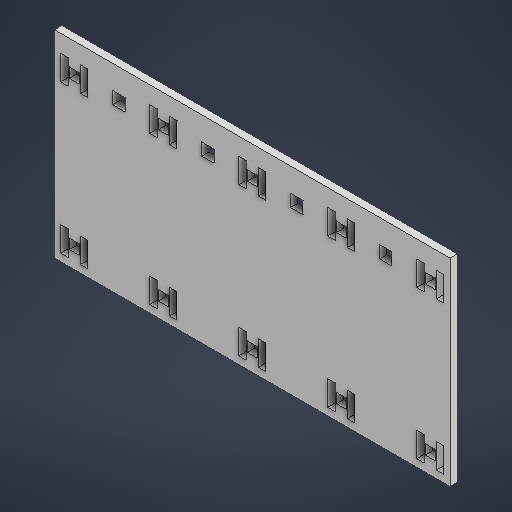
# Autodesk Inventor part: techo
Saved by Autodesk Inventor 2026 (Build 300175000, 175)
## iProperties
Created: 2026-05-15
Part Number: techo
Material: Generic
Document SubType Name: Modeling
Designer: juana
Density: 1 g/cm^3
Appearance: Default
Author: juana
Autodesk Inventor part; units mm, degrees
ref_plane "YZ Plane" through (0, 0, 0) normal (1, 0, 0) x (0, 1, 0)
ref_plane "XZ Plane" through (0, 0, 0) normal (0, 1, 0) x (-1, 0, 0)
ref_plane "XY Plane" through (0, 0, 0) normal (0, 0, 1) x (1, 0, 0)
sketch "Sketch1" plane through (0, 0, 0) normal (0, 0, 1) x (1, 0, 0)
  line L0 (0, 0) -> (160, 0)
  line L1 (160, 0) -> (160, 80)
  line L2 (160, 80) -> (0, 80)
  line L3 (0, 80) -> (0, 0)
  line L4 (2.5, 13) -> (5.5, 13)
  line L5 (5.5, 13) -> (5.5, 3)
  line L6 (5.5, 3) -> (2.5, 3)
  line L7 (2.5, 3) -> (2.5, 13)
  line L8 (10.5, 13) -> (13.5, 13)
  line L9 (13.5, 13) -> (13.5, 3)
  line L10 (13.5, 3) -> (10.5, 3)
  line L11 (10.5, 3) -> (10.5, 13)
  line L12 (0, 40) -> (160, 40) construction
  line L13 (80, 80) -> (80, 0) construction
  line L14 (0, 0) -> (0, 80)
  line L15 (2.5, 77) -> (2.5, 67) construction
  line L16 (13.5, 77) -> (10.5, 77)
  line L17 (157.5, 13) -> (154.5, 13)
  line L18 (154.5, 13) -> (154.5, 3)
  line L19 (154.5, 3) -> (157.5, 3)
  line L20 (157.5, 3) -> (157.5, 13)
  line L21 (149.5, 13) -> (146.5, 13)
  line L22 (146.5, 13) -> (146.5, 3)
  line L23 (146.5, 3) -> (149.5, 3)
  line L24 (149.5, 3) -> (149.5, 13)
  line L25 (2.5, 77) -> (157.5, 77) construction
  line L26 (157.5, 77) -> (157.5, 3) construction
  line L27 (157.5, 3) -> (2.5, 3) construction
  line L28 (2.5, 3) -> (2.5, 77) construction
  line L29 (5.5, 13) -> (5.5, 3)
  line L30 (6, 6) -> (10, 6)
  line L31 (10, 6) -> (10, 10)
  line L32 (10, 10) -> (6, 10)
  line L33 (6, 10) -> (6, 6)
  line L34 (23.49, 65.49) -> (28.51, 65.49)
  line L35 (28.51, 65.49) -> (28.51, 70.51)
  line L36 (28.51, 70.51) -> (23.49, 70.51)
  line L37 (23.49, 70.51) -> (23.49, 65.49)
  line L38 (59.49, 65.49) -> (64.51, 65.49)
  line L39 (64.51, 70.51) -> (59.49, 70.51)
  line L40 (64.51, 65.49) -> (64.51, 70.51)
  line L41 (59.49, 70.51) -> (59.49, 65.49)
  line L42 (95.49, 65.49) -> (100.51, 65.49)
  line L43 (100.51, 70.51) -> (95.49, 70.51)
  line L44 (100.51, 65.49) -> (100.51, 70.51)
  line L45 (95.49, 70.51) -> (95.49, 65.49)
  line L46 (131.49, 65.49) -> (136.51, 65.49)
  line L47 (136.51, 70.51) -> (131.49, 70.51)
  line L48 (136.51, 65.49) -> (136.51, 70.51)
  line L49 (131.49, 70.51) -> (131.49, 65.49)
  line L50 (2.5, 73) -> (5.5, 73)
  line L51 (5.5, 73) -> (5.5, 63)
  line L52 (5.5, 63) -> (2.5, 63)
  line L53 (2.5, 63) -> (2.5, 73)
  line L54 (6, 70) -> (10, 70)
  line L55 (10, 70) -> (10, 66)
  line L56 (10, 66) -> (6, 66)
  line L57 (6, 66) -> (6, 70)
  line L58 (10.5, 73) -> (13.5, 73)
  line L59 (13.5, 73) -> (13.5, 63)
  line L60 (13.5, 63) -> (10.5, 63)
  line L61 (10.5, 63) -> (10.5, 73)
  line L62 (157.5, 77) -> (157.5, 67) construction
  line L63 (157.5, 3) -> (157.5, 77) construction
  line L64 (157.5, 73) -> (154.5, 73)
  line L65 (154.5, 73) -> (154.5, 63)
  line L66 (154.5, 63) -> (157.5, 63)
  line L67 (157.5, 63) -> (157.5, 73)
  line L68 (154, 70) -> (150, 70)
  line L69 (150, 70) -> (150, 66)
  line L70 (150, 66) -> (154, 66)
  line L71 (154, 66) -> (154, 70)
  line L72 (149.5, 73) -> (146.5, 73)
  line L73 (146.5, 73) -> (146.5, 63)
  line L74 (146.5, 63) -> (149.5, 63)
  line L75 (149.5, 63) -> (149.5, 73)
  line L76 (154.5, 13) -> (154.5, 3)
  line L77 (150, 6) -> (150, 10)
  line L78 (150, 10) -> (154, 10)
  line L79 (154, 10) -> (154, 6)
  line L80 (154, 6) -> (150, 6)
  line L81 (38.5, 77) -> (38.5, 67) construction
  line L82 (46, 70) -> (46, 66)
  line L83 (46.5, 63) -> (46.5, 73)
  line L84 (42, 70) -> (46, 70)
  line L85 (42, 66) -> (42, 70)
  line L86 (41.5, 73) -> (41.5, 63)
  line L87 (38.5, 73) -> (41.5, 73)
  line L88 (38.5, 63) -> (38.5, 73)
  line L89 (38.5, 3) -> (38.5, 77) construction
  line L90 (41.5, 63) -> (38.5, 63)
  line L91 (46, 66) -> (42, 66)
  line L92 (49.5, 63) -> (46.5, 63)
  line L93 (49.5, 73) -> (49.5, 63)
  line L94 (46.5, 73) -> (49.5, 73)
  line L95 (74.5, 77) -> (74.5, 67) construction
  line L96 (82, 70) -> (82, 66)
  line L97 (82.5, 63) -> (82.5, 73)
  line L98 (78, 70) -> (82, 70)
  line L99 (78, 66) -> (78, 70)
  line L100 (77.5, 73) -> (77.5, 63)
  line L101 (74.5, 73) -> (77.5, 73)
  line L102 (74.5, 63) -> (74.5, 73)
  line L103 (74.5, 3) -> (74.5, 77) construction
  line L104 (77.5, 63) -> (74.5, 63)
  line L105 (82, 66) -> (78, 66)
  line L106 (85.5, 63) -> (82.5, 63)
  line L107 (85.5, 73) -> (85.5, 63)
  line L108 (82.5, 73) -> (85.5, 73)
  line L109 (110.5, 77) -> (110.5, 67) construction
  line L110 (118, 70) -> (118, 66)
  line L111 (118.5, 63) -> (118.5, 73)
  line L112 (114, 70) -> (118, 70)
  line L113 (114, 66) -> (114, 70)
  line L114 (113.5, 73) -> (113.5, 63)
  line L115 (110.5, 73) -> (113.5, 73)
  line L116 (110.5, 63) -> (110.5, 73)
  line L117 (110.5, 3) -> (110.5, 77) construction
  line L118 (113.5, 63) -> (110.5, 63)
  line L119 (118, 66) -> (114, 66)
  line L120 (121.5, 63) -> (118.5, 63)
  line L121 (121.5, 73) -> (121.5, 63)
  line L122 (118.5, 73) -> (121.5, 73)
  line L123 (146.5, 77) -> (146.5, 67) construction
  line L124 (154, 70) -> (154, 66)
  line L125 (154.5, 63) -> (154.5, 73)
  line L126 (150, 70) -> (154, 70)
  line L127 (150, 66) -> (150, 70)
  line L128 (149.5, 73) -> (149.5, 63)
  line L129 (146.5, 73) -> (149.5, 73)
  line L130 (146.5, 63) -> (146.5, 73)
  line L131 (146.5, 3) -> (146.5, 77) construction
  line L132 (149.5, 63) -> (146.5, 63)
  line L133 (154, 66) -> (150, 66)
  line L134 (157.5, 63) -> (154.5, 63)
  line L135 (157.5, 73) -> (157.5, 63)
  line L136 (154.5, 73) -> (157.5, 73)
  line L137 (2.5, 17) -> (2.5, 7) construction
  line L138 (10, 10) -> (10, 6)
  line L139 (10.5, 3) -> (10.5, 13)
  line L140 (6, 10) -> (10, 10)
  line L141 (6, 6) -> (6, 10)
  line L142 (5.5, 13) -> (5.5, 3)
  line L143 (2.5, 13) -> (5.5, 13)
  line L144 (2.5, 3) -> (2.5, 13)
  line L145 (2.5, -57) -> (2.5, 17) construction
  line L146 (5.5, 3) -> (2.5, 3)
  line L147 (10, 6) -> (6, 6)
  line L148 (13.5, 3) -> (10.5, 3)
  line L149 (13.5, 13) -> (13.5, 3)
  line L150 (10.5, 13) -> (13.5, 13)
  line L151 (38.5, 17) -> (38.5, 7) construction
  line L152 (46, 10) -> (46, 6)
  line L153 (46.5, 3) -> (46.5, 13)
  line L154 (42, 10) -> (46, 10)
  line L155 (42, 6) -> (42, 10)
  line L156 (41.5, 13) -> (41.5, 3)
  line L157 (38.5, 13) -> (41.5, 13)
  line L158 (38.5, 3) -> (38.5, 13)
  line L159 (38.5, -57) -> (38.5, 17) construction
  line L160 (41.5, 3) -> (38.5, 3)
  line L161 (46, 6) -> (42, 6)
  line L162 (49.5, 3) -> (46.5, 3)
  line L163 (49.5, 13) -> (49.5, 3)
  line L164 (46.5, 13) -> (49.5, 13)
  line L165 (74.5, 17) -> (74.5, 7) construction
  line L166 (82, 10) -> (82, 6)
  line L167 (82.5, 3) -> (82.5, 13)
  line L168 (78, 10) -> (82, 10)
  line L169 (78, 6) -> (78, 10)
  line L170 (77.5, 13) -> (77.5, 3)
  line L171 (74.5, 13) -> (77.5, 13)
  line L172 (74.5, 3) -> (74.5, 13)
  line L173 (74.5, -57) -> (74.5, 17) construction
  line L174 (77.5, 3) -> (74.5, 3)
  line L175 (82, 6) -> (78, 6)
  line L176 (85.5, 3) -> (82.5, 3)
  line L177 (85.5, 13) -> (85.5, 3)
  line L178 (82.5, 13) -> (85.5, 13)
  line L179 (110.5, 17) -> (110.5, 7) construction
  line L180 (118, 10) -> (118, 6)
  line L181 (118.5, 3) -> (118.5, 13)
  line L182 (114, 10) -> (118, 10)
  line L183 (114, 6) -> (114, 10)
  line L184 (113.5, 13) -> (113.5, 3)
  line L185 (110.5, 13) -> (113.5, 13)
  line L186 (110.5, 3) -> (110.5, 13)
  line L187 (110.5, -57) -> (110.5, 17) construction
  line L188 (113.5, 3) -> (110.5, 3)
  line L189 (118, 6) -> (114, 6)
  line L190 (121.5, 3) -> (118.5, 3)
  line L191 (121.5, 13) -> (121.5, 3)
  line L192 (118.5, 13) -> (121.5, 13)
  line L193 (146.5, 17) -> (146.5, 7) construction
  line L194 (154, 10) -> (154, 6)
  line L195 (154.5, 3) -> (154.5, 13)
  line L196 (150, 10) -> (154, 10)
  line L197 (150, 6) -> (150, 10)
  line L198 (149.5, 13) -> (149.5, 3)
  line L199 (146.5, 13) -> (149.5, 13)
  line L200 (146.5, 3) -> (146.5, 13)
  line L201 (146.5, -57) -> (146.5, 17) construction
  line L202 (149.5, 3) -> (146.5, 3)
  line L203 (154, 6) -> (150, 6)
  line L204 (157.5, 3) -> (154.5, 3)
  line L205 (157.5, 13) -> (157.5, 3)
  line L206 (154.5, 13) -> (157.5, 13)
  point P0 (23.49, 68)
  point P1 (26, 70.51)
  point P2 (62, 70.51)
  point P3 (59.49, 68)
  point P4 (98, 70.51)
  point P5 (95.49, 68)
  point P6 (134, 70.51)
  point P7 (131.49, 68)
  point P8 (2.5, 72)
  point P9 (5.5, 68)
  point P10 (6, 68)
  point P11 (8, 66)
  point P12 (8, 10)
  point P13 (157.5, 72)
  point P14 (154.5, 68)
  point P15 (154, 68)
  point P16 (152, 66)
  point P17 (38.5, 72)
  point P18 (44, 66)
  point P19 (42, 68)
  point P20 (41.5, 68)
  point P21 (74.5, 72)
  point P22 (80, 66)
  point P23 (78, 68)
  point P24 (77.5, 68)
  point P25 (110.5, 72)
  point P26 (116, 66)
  point P27 (114, 68)
  point P28 (113.5, 68)
  point P29 (146.5, 72)
  point P30 (152, 66)
  point P31 (150, 68)
  point P32 (149.5, 68)
  point P33 (2.5, 12)
  point P34 (8, 6)
  point P35 (6, 8)
  point P36 (5.5, 8)
  point P37 (38.5, 12)
  point P38 (44, 6)
  point P39 (42, 8)
  point P40 (41.5, 8)
  point P41 (74.5, 12)
  point P42 (80, 6)
  point P43 (78, 8)
  point P44 (77.5, 8)
  point P45 (110.5, 12)
  point P46 (116, 6)
  point P47 (114, 8)
  point P48 (113.5, 8)
  point P49 (146.5, 12)
  point P50 (152, 6)
  point P51 (150, 8)
  point P52 (149.5, 8)
  dimension "d0" = 80
  dimension "d1" = 160
  dimension "d2" = 3
  dimension "d3" = 2.5
  dimension "d4" = 3
  dimension "d5" = 10
  dimension "d6" = 5
  dimension "d11" = 5.02
  dimension "d12" = 5.02
  dimension "d13" = 23.5
  dimension "d16" = 36
  dimension "d23" = 70
  dimension "d24" = 3
  dimension "d25" = 3
  dimension "d26" = 0.5
  dimension "d27" = 0.5
  dimension "d30" = 36
  dimension "d33" = 60
  constraints: 414 end point, 36 symmetric about line, 16 parallel, 11 midpoint, 11 point on line, 10 horizontal, 8 equal length, 8 perpendicular, 4 horizontal alignment, 3 vertical alignment, 1 vertical, 327 other
  measures "d0" distance of L0.end L1.end
  measures "d1" distance of L0.start L0.end
  measures "d2" distance of L4.start L4.end
  measures "d3" distance between parallel lines of L3 L7
  measures "d4" distance between parallel lines of L0 L6
  measures "d5" distance of L4.end L5.end
  measures "d6" distance between parallel lines of L11 L5
  measures "d11" distance of L35.end L36.end
  measures "d12" distance of L34.end L35.end
  measures "d13" distance from line of L28 point (26, 70.51)
  measures "d16" distance of L34.end L38.end
  measures "d23" distance from line of L6.end L50
  measures "d24" distance between parallel lines of L8 L32
  measures "d25" distance between parallel lines of L27 L30
  measures "d26" distance between parallel lines of L11 L31
  measures "d27" distance between parallel lines of L5 L33
  measures "d30" distance of L15.end L81.end
  measures "d33" distance of L15.end L137.end
extrude "Extrusion1" add sketch "Sketch1" along normal blind 3
body "Solid1"
